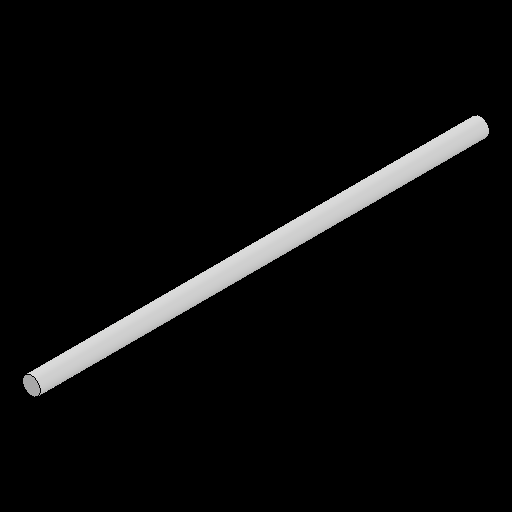
# Autodesk Inventor part: 大軸
Saved by Autodesk Inventor 2022 (Build 260153000, 153)
## iProperties
Created: 2021-07-07
Part Number: 大軸
Material: 一般
Document SubType Name: Modeling
Designer: nrz71
Density: 1 g/cm^3
Appearance: 既定
Author: nrz71
Autodesk Inventor part; units mm, degrees
ref_plane "YZ Plane" through (0, 0, 0) normal (1, 0, 0) x (0, 1, 0)
ref_plane "XZ Plane" through (0, 0, 0) normal (0, 1, 0) x (-1, 0, 0)
ref_plane "XY Plane" through (0, 0, 0) normal (0, 0, 1) x (1, 0, 0)
sketch "スケッチ1" plane through (0, 0, 0) normal (0, 0, 1) x (1, 0, 0)
  circle A0 centre (0, 0) radius 3
  dimension "d0" = 6
  constraints: 1 centre point, 1 coincident
  measures "d0" diameter of A0
ref_plane "作業平面1" through (0, 0, -150) normal (0, 0, -1) x (0, 1, 0)
extrude "押し出し1" add sketch "スケッチ1" against normal up to surface (150 mm away)
